camera_mount (Autodesk Fusion 360 design; units mm, degrees)
Autodesk Fusion 360 part; units mm, degrees
sketch "Sketch1" plane through (0, 0, 0) normal (1, 0, 0) x (0, 1, 0)
  circle A0 centre (0, 0) radius 27.5
  line L0 (-22, 16.5) -> (22, 16.5)
  circle A1 centre (0, 0) radius 35
  line L1 (27.5, 0) -> (-27.5, 0)
  dimension "d1" = 55
  dimension "d2" = 44
  dimension "d3" = 70
  constraint coincident A0.centre A1.centre
  constraint coincident A0 L0.start
  constraint coincident A0 L0.end
  constraint horizontal L0
  constraint coincident A0 L1.start
  constraint coincident A0 L1.end
  constraint horizontal L1
  constraint coincident A0.centre L1
  measures "d1" diameter of A0
  measures "d2" distance of L0.start L0.end
  measures "d3" diameter of A1
sketch "Sketch2" plane through (0, 0, 0) normal (1, 0, 0) x (0, 1, 0)
  line L0 (-17.5, 25) -> (17.5, 25)
  line L1 (17.5, 25) -> (17.5, -25)
  line L2 (17.5, -25) -> (-17.5, -25)
  line L3 (-17.5, -25) -> (-17.5, 25)
  line L4 (0, 0) -> (0, 25)
  line L5 (0, 0) -> (17.5, 0)
  dimension "d4" = 35
  dimension "d5" = 50
  constraint horizontal L0
  constraint vertical L1
  constraint horizontal L2
  constraint vertical L3
  constraint coincident L4.start L5.start
  constraint coincident L0 L4.end
  constraint perpendicular L0 L4
  constraint midpoint L0 L4.end
  constraint coincident L1 L5.end
  constraint perpendicular L1 L5
  constraint midpoint L1 L5.end
  measures "d4" distance of L0.start L0.end
  measures "d5" distance of L0.end L1.end
extrude "Extrude1" add sketch "Sketch2" against normal blind 23
sketch "Sketch3" plane through (-23, 0, 0) normal (-1, 0, 0) x (0, -1, 0)
  line L0 (-17.5, -25) -> (17.5, -25)
  line L1 (17.5, -25) -> (17.5, 25)
  line L2 (17.5, 25) -> (-17.5, 25)
  line L3 (-17.5, 25) -> (-17.5, -25)
  line L4 (-13.5, 25) -> (13.5, 25)
  line L5 (13.5, 25) -> (13.5, -25)
  line L6 (13.5, -25) -> (-13.5, -25)
  line L7 (-13.5, -25) -> (-13.5, 25)
  line L8 (0, 0) -> (0, 25)
  dimension "d8" = 27
  constraint horizontal L4
  constraint vertical L5
  constraint horizontal L6
  constraint vertical L7
  constraint coincident L0 L5.end
  constraint coincident L2 L4.start
  constraint coincident L8.start origin
  constraint midpoint L2 L8.end
  constraint midpoint L4 L8.end
  measures "d8" distance of L4.start L4.end
extrude "Extrude2" cut sketch "Sketch3" against normal blind 15 contours L0 L2 L4 L5 L6 L7
extrude "Extrude3" add sketch "Sketch1" along normal blind 9 contours A0 L0 L1 | A0 L1 | A0 L0 | A1
extrude "Extrude4" cut sketch "Sketch1" along normal blind 6.5 contours A0 L0 L1 | A0 L1
sketch "Sketch5" plane through (0, 0, 0) normal (0, 0, 1) x (1, 0, 0)
extrude "Extrude5" add sketch "Sketch1" against normal blind 2 contours A0 L0 L1 | A0 L1 | A0 L0 | A1
sketch "Sketch6" plane through (9, 0, 0) normal (1, 0, 0) x (0, 1, 0)
  circle A0 centre (0, 0) radius 35
  line L0 (-27, 0) -> (27.5, 0)
  line L1 (27.5, 0) -> (27.5, 40)
  line L2 (27.5, 40) -> (-27, 40)
  line L3 (-27, 40) -> (-27, 0)
  point P0 (27.5, 0)
  dimension "d17" = 40
  constraint horizontal L0
  constraint vertical L1
  constraint horizontal L2
  constraint vertical L3
  constraint coincident P0 L0.end
  measures "d17" distance of P0 L1.end
extrude "Extrude6" cut sketch "Sketch6" against normal blind 9 contours A0 L0 L1 L3 | A0 L1 L2 L3 picked at (0.2995, 11.6659)
sketch "Sketch7" plane through (0, 0, 0) normal (1, 0, 0) x (0, 1, 0)
  circle A0 centre (0, 0) radius 10
  dimension "d20" = 20
  constraint coincident A0.centre origin
  measures "d20" diameter of A0
extrude "Extrude7" cut sketch "Sketch7" along normal blind 25
